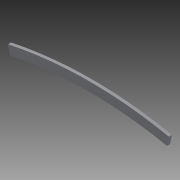
# Autodesk Inventor part: nd-9
Saved by Autodesk Inventor 2015 (Build 190159000, 159)
## iProperties
Created: 2014-07-02
Part Number: nd-9
Material: Generic
Document SubType Name: Modeling
Designer: peter
Density: 1 g/cm^3
Appearance: Default
Author: peter
Autodesk Inventor part; units mm, degrees
ref_plane "YZ Plane" through (0, 0, 0) normal (1, 0, 0) x (0, 1, 0)
ref_plane "XZ Plane" through (0, 0, 0) normal (0, 1, 0) x (-1, 0, 0)
ref_plane "XY Plane" through (0, 0, 0) normal (0, 0, 1) x (1, 0, 0)
sketch "Sketch1" plane through (0, 0, 0) normal (0, 0, 1) x (1, 0, 0)
  arc A0 (1008.5687, 58.1213) -> (0.1285, 55.9387) centre (509.5261, -2335.1519) ccw
  line L0 (0.1285, 55.9387) -> (12.0365, 0.0431)
  arc A1 (996.9027, 2.1746) -> (12.0365, 0.0431) centre (509.5261, -2335.1524) ccw
  line L1 (996.9027, 2.1746) -> (1008.5687, 58.1213)
  point P0 (0, 0)
  constraints: 4 end point, 4 point on circle, 2 centre point
extrude "Extrusion1" add sketch "Sketch1" along normal blind 19.05
body "Solid1"
